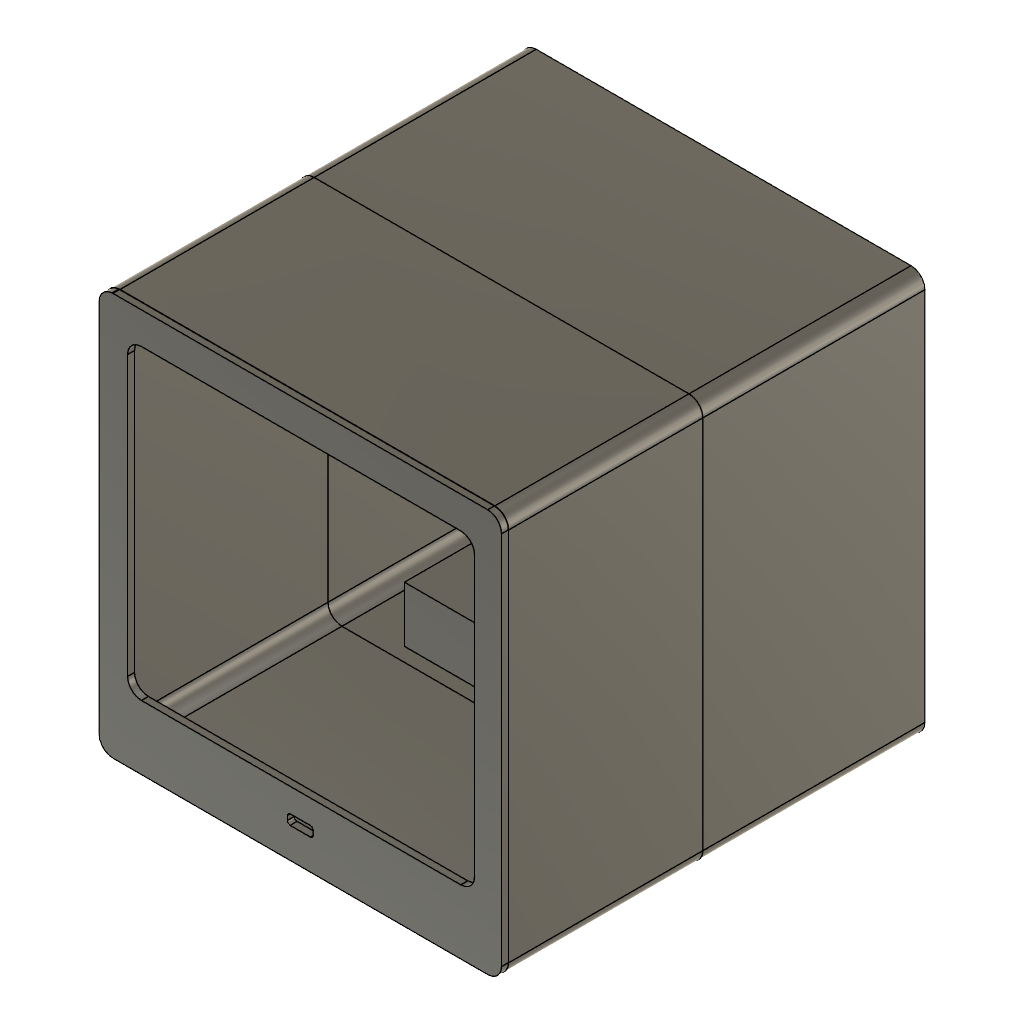
Fume Absorber (Autodesk Fusion 360 design; units mm, degrees)
part number: 2026-09-16-20-58-32-187
Autodesk Fusion 360 part; units mm, degrees
note: some values were not read from the file. Set by a fixed rule: which sketch regions a step uses.
(part 1 of 2)
sketch "Sketch2" plane through (0, 0, 0) normal (0, 1, 0) x (1, 0, 0)
  line L0 (-57.9957, -145.0372) -> (77.0043, -145.0372)
  line L1 (82.0043, -140.0372) -> (82.0043, -5.0372)
  line L2 (77.0043, -0.0372) -> (-57.9957, -0.0372)
  line L3 (-62.9957, -5.0372) -> (-62.9957, -140.0372)
  arc A0 (-62.9957, -140.0372) -> (-57.9957, -145.0372) centre (-57.9957, -140.0372) ccw
  arc A1 (77.0043, -145.0372) -> (82.0043, -140.0372) centre (77.0043, -140.0372) ccw
  arc A2 (82.0043, -5.0372) -> (77.0043, -0.0372) centre (77.0043, -5.0372) ccw
  arc A3 (-57.9957, -0.0372) -> (-62.9957, -5.0372) centre (-57.9957, -5.0372) ccw
  line L4 (-47.9957, -135.0372) -> (67.0043, -135.0372)
  line L5 (72.0043, -130.0372) -> (72.0043, -15.0372)
  line L6 (67.0043, -10.0372) -> (-47.9957, -10.0372)
  line L7 (-52.9957, -15.0372) -> (-52.9957, -130.0372)
  arc A4 (-52.9957, -130.0372) -> (-47.9957, -135.0372) centre (-47.9957, -130.0372) ccw
  arc A5 (67.0043, -135.0372) -> (72.0043, -130.0372) centre (67.0043, -130.0372) ccw
  arc A6 (72.0043, -15.0372) -> (67.0043, -10.0372) centre (67.0043, -15.0372) ccw
  arc A7 (-47.9957, -10.0372) -> (-52.9957, -15.0372) centre (-47.9957, -15.0372) ccw
  circle A8 centre (3.6938, -81.3062) radius 2.5
  circle A9 centre (10.5725, -75.1918) radius 2.5
  circle A10 centre (-66.3062, -141.3062) radius 2.5
  circle A11 centre (-59.4275, -135.1918) radius 2.5
  circle A12 centre (-59.3062, -141.3062) radius 2.5
  circle A13 centre (-52.4275, -135.1918) radius 2.5
  circle A14 centre (-52.3062, -141.3062) radius 2.5
  circle A15 centre (-45.4275, -135.1918) radius 2.5
  circle A16 centre (-45.3062, -141.3062) radius 2.5
  circle A17 centre (-38.4275, -135.1918) radius 2.5
  circle A18 centre (-38.3062, -141.3062) radius 2.5
  circle A19 centre (-31.4275, -135.1918) radius 2.5
  circle A20 centre (-31.3062, -141.3062) radius 2.5
  circle A21 centre (-24.4275, -135.1918) radius 2.5
  circle A22 centre (-24.3062, -141.3062) radius 2.5
  circle A23 centre (-17.4275, -135.1918) radius 2.5
  circle A24 centre (-17.3062, -141.3062) radius 2.5
  circle A25 centre (-10.4275, -135.1918) radius 2.5
  circle A26 centre (-10.3062, -141.3062) radius 2.5
  circle A27 centre (-3.4275, -135.1918) radius 2.5
  circle A28 centre (-3.3062, -141.3062) radius 2.5
  circle A29 centre (3.5725, -135.1918) radius 2.5
  circle A30 centre (3.6938, -141.3062) radius 2.5
  circle A31 centre (10.5725, -135.1918) radius 2.5
  circle A32 centre (10.6938, -141.3062) radius 2.5
  circle A33 centre (17.5725, -135.1918) radius 2.5
  circle A34 centre (17.6938, -141.3062) radius 2.5
  circle A35 centre (24.5725, -135.1918) radius 2.5
  circle A36 centre (24.6938, -141.3062) radius 2.5
  circle A37 centre (31.5725, -135.1918) radius 2.5
  circle A38 centre (31.6938, -141.3062) radius 2.5
  circle A39 centre (38.5725, -135.1918) radius 2.5
  circle A40 centre (38.6938, -141.3062) radius 2.5
  circle A41 centre (45.5725, -135.1918) radius 2.5
  circle A42 centre (45.6938, -141.3062) radius 2.5
  circle A43 centre (52.5725, -135.1918) radius 2.5
  circle A44 centre (52.6938, -141.3062) radius 2.5
  circle A45 centre (59.5725, -135.1918) radius 2.5
  circle A46 centre (59.6938, -141.3062) radius 2.5
  circle A47 centre (66.5725, -135.1918) radius 2.5
  circle A48 centre (66.6938, -141.3062) radius 2.5
  circle A49 centre (73.5725, -135.1918) radius 2.5
  circle A50 centre (73.6938, -141.3062) radius 2.5
  circle A51 centre (80.5725, -135.1918) radius 2.5
  circle A52 centre (-66.3062, -135.3062) radius 2.5
  circle A53 centre (-59.4275, -129.1918) radius 2.5
  circle A54 centre (-59.3062, -135.3062) radius 2.5
  circle A55 centre (-52.4275, -129.1918) radius 2.5
  circle A56 centre (-52.3062, -135.3062) radius 2.5
  circle A57 centre (-45.4275, -129.1918) radius 2.5
  circle A58 centre (-45.3062, -135.3062) radius 2.5
  circle A59 centre (-38.4275, -129.1918) radius 2.5
  circle A60 centre (-38.3062, -135.3062) radius 2.5
  circle A61 centre (-31.4275, -129.1918) radius 2.5
  circle A62 centre (-31.3062, -135.3062) radius 2.5
  circle A63 centre (-24.4275, -129.1918) radius 2.5
  circle A64 centre (-24.3062, -135.3062) radius 2.5
  circle A65 centre (-17.4275, -129.1918) radius 2.5
  circle A66 centre (-17.3062, -135.3062) radius 2.5
  circle A67 centre (-10.4275, -129.1918) radius 2.5
  circle A68 centre (-10.3062, -135.3062) radius 2.5
  circle A69 centre (-3.4275, -129.1918) radius 2.5
  circle A70 centre (-3.3062, -135.3062) radius 2.5
  circle A71 centre (3.5725, -129.1918) radius 2.5
  circle A72 centre (3.6938, -135.3062) radius 2.5
  circle A73 centre (10.5725, -129.1918) radius 2.5
  circle A74 centre (10.6938, -135.3062) radius 2.5
  circle A75 centre (17.5725, -129.1918) radius 2.5
  circle A76 centre (17.6938, -135.3062) radius 2.5
  circle A77 centre (24.5725, -129.1918) radius 2.5
  circle A78 centre (24.6938, -135.3062) radius 2.5
  circle A79 centre (31.5725, -129.1918) radius 2.5
  circle A80 centre (31.6938, -135.3062) radius 2.5
  circle A81 centre (38.5725, -129.1918) radius 2.5
  circle A82 centre (38.6938, -135.3062) radius 2.5
  circle A83 centre (45.5725, -129.1918) radius 2.5
  circle A84 centre (45.6938, -135.3062) radius 2.5
  circle A85 centre (52.5725, -129.1918) radius 2.5
  circle A86 centre (52.6938, -135.3062) radius 2.5
  circle A87 centre (59.5725, -129.1918) radius 2.5
  circle A88 centre (59.6938, -135.3062) radius 2.5
  circle A89 centre (66.5725, -129.1918) radius 2.5
  circle A90 centre (66.6938, -135.3062) radius 2.5
  circle A91 centre (73.5725, -129.1918) radius 2.5
  circle A92 centre (73.6938, -135.3062) radius 2.5
  circle A93 centre (80.5725, -129.1918) radius 2.5
  circle A94 centre (-66.3062, -129.3062) radius 2.5
  circle A95 centre (-59.4275, -123.1918) radius 2.5
  circle A96 centre (-59.3062, -129.3062) radius 2.5
  circle A97 centre (-52.4275, -123.1918) radius 2.5
  circle A98 centre (-52.3062, -129.3062) radius 2.5
  circle A99 centre (-45.4275, -123.1918) radius 2.5
  circle A100 centre (-45.3062, -129.3062) radius 2.5
  circle A101 centre (-38.4275, -123.1918) radius 2.5
  circle A102 centre (-38.3062, -129.3062) radius 2.5
  circle A103 centre (-31.4275, -123.1918) radius 2.5
  circle A104 centre (-31.3062, -129.3062) radius 2.5
  circle A105 centre (-24.4275, -123.1918) radius 2.5
  circle A106 centre (-24.3062, -129.3062) radius 2.5
  circle A107 centre (-17.4275, -123.1918) radius 2.5
  circle A108 centre (-17.3062, -129.3062) radius 2.5
  circle A109 centre (-10.4275, -123.1918) radius 2.5
  circle A110 centre (-10.3062, -129.3062) radius 2.5
  circle A111 centre (-3.4275, -123.1918) radius 2.5
  circle A112 centre (-3.3062, -129.3062) radius 2.5
  circle A113 centre (3.5725, -123.1918) radius 2.5
  circle A114 centre (3.6938, -129.3062) radius 2.5
  circle A115 centre (10.5725, -123.1918) radius 2.5
  circle A116 centre (10.6938, -129.3062) radius 2.5
  circle A117 centre (17.5725, -123.1918) radius 2.5
  circle A118 centre (17.6938, -129.3062) radius 2.5
  circle A119 centre (24.5725, -123.1918) radius 2.5
  circle A120 centre (24.6938, -129.3062) radius 2.5
  circle A121 centre (31.5725, -123.1918) radius 2.5
  circle A122 centre (31.6938, -129.3062) radius 2.5
  circle A123 centre (38.5725, -123.1918) radius 2.5
  circle A124 centre (38.6938, -129.3062) radius 2.5
  circle A125 centre (45.5725, -123.1918) radius 2.5
  circle A126 centre (45.6938, -129.3062) radius 2.5
  circle A127 centre (52.5725, -123.1918) radius 2.5
  circle A128 centre (52.6938, -129.3062) radius 2.5
  circle A129 centre (59.5725, -123.1918) radius 2.5
  circle A130 centre (59.6938, -129.3062) radius 2.5
  circle A131 centre (66.5725, -123.1918) radius 2.5
  circle A132 centre (66.6938, -129.3062) radius 2.5
  circle A133 centre (73.5725, -123.1918) radius 2.5
  circle A134 centre (73.6938, -129.3062) radius 2.5
  circle A135 centre (80.5725, -123.1918) radius 2.5
  circle A136 centre (-66.3062, -123.3062) radius 2.5
  circle A137 centre (-59.4275, -117.1918) radius 2.5
  circle A138 centre (-59.3062, -123.3062) radius 2.5
  circle A139 centre (-52.4275, -117.1918) radius 2.5
  circle A140 centre (-52.3062, -123.3062) radius 2.5
  circle A141 centre (-45.4275, -117.1918) radius 2.5
  circle A142 centre (-45.3062, -123.3062) radius 2.5
  circle A143 centre (-38.4275, -117.1918) radius 2.5
  circle A144 centre (-38.3062, -123.3062) radius 2.5
  circle A145 centre (-31.4275, -117.1918) radius 2.5
  circle A146 centre (-31.3062, -123.3062) radius 2.5
  circle A147 centre (-24.4275, -117.1918) radius 2.5
  circle A148 centre (-24.3062, -123.3062) radius 2.5
  circle A149 centre (-17.4275, -117.1918) radius 2.5
  circle A150 centre (-17.3062, -123.3062) radius 2.5
  circle A151 centre (-10.4275, -117.1918) radius 2.5
  circle A152 centre (-10.3062, -123.3062) radius 2.5
  circle A153 centre (-3.4275, -117.1918) radius 2.5
  circle A154 centre (-3.3062, -123.3062) radius 2.5
  circle A155 centre (3.5725, -117.1918) radius 2.5
  circle A156 centre (3.6938, -123.3062) radius 2.5
  circle A157 centre (10.5725, -117.1918) radius 2.5
  circle A158 centre (10.6938, -123.3062) radius 2.5
  circle A159 centre (17.5725, -117.1918) radius 2.5
  circle A160 centre (17.6938, -123.3062) radius 2.5
  circle A161 centre (24.5725, -117.1918) radius 2.5
  circle A162 centre (24.6938, -123.3062) radius 2.5
  circle A163 centre (31.5725, -117.1918) radius 2.5
  circle A164 centre (31.6938, -123.3062) radius 2.5
  circle A165 centre (38.5725, -117.1918) radius 2.5
  circle A166 centre (38.6938, -123.3062) radius 2.5
  circle A167 centre (45.5725, -117.1918) radius 2.5
  circle A168 centre (45.6938, -123.3062) radius 2.5
  circle A169 centre (52.5725, -117.1918) radius 2.5
  circle A170 centre (52.6938, -123.3062) radius 2.5
  circle A171 centre (59.5725, -117.1918) radius 2.5
  circle A172 centre (59.6938, -123.3062) radius 2.5
  circle A173 centre (66.5725, -117.1918) radius 2.5
  circle A174 centre (66.6938, -123.3062) radius 2.5
  circle A175 centre (73.5725, -117.1918) radius 2.5
  circle A176 centre (73.6938, -123.3062) radius 2.5
  circle A177 centre (80.5725, -117.1918) radius 2.5
  circle A178 centre (-66.3062, -117.3062) radius 2.5
  circle A179 centre (-59.4275, -111.1918) radius 2.5
  circle A180 centre (-59.3062, -117.3062) radius 2.5
  circle A181 centre (-52.4275, -111.1918) radius 2.5
  circle A182 centre (-52.3062, -117.3062) radius 2.5
  circle A183 centre (-45.4275, -111.1918) radius 2.5
  circle A184 centre (-45.3062, -117.3062) radius 2.5
  circle A185 centre (-38.4275, -111.1918) radius 2.5
  circle A186 centre (-38.3062, -117.3062) radius 2.5
  circle A187 centre (-31.4275, -111.1918) radius 2.5
  circle A188 centre (-31.3062, -117.3062) radius 2.5
  circle A189 centre (-24.4275, -111.1918) radius 2.5
  circle A190 centre (-24.3062, -117.3062) radius 2.5
  circle A191 centre (-17.4275, -111.1918) radius 2.5
  circle A192 centre (-17.3062, -117.3062) radius 2.5
  circle A193 centre (-10.4275, -111.1918) radius 2.5
  circle A194 centre (-10.3062, -117.3062) radius 2.5
  circle A195 centre (-3.4275, -111.1918) radius 2.5
  circle A196 centre (-3.3062, -117.3062) radius 2.5
  circle A197 centre (3.5725, -111.1918) radius 2.5
  circle A198 centre (3.6938, -117.3062) radius 2.5
  circle A199 centre (10.5725, -111.1918) radius 2.5
  circle A200 centre (10.6938, -117.3062) radius 2.5
  circle A201 centre (17.5725, -111.1918) radius 2.5
  circle A202 centre (17.6938, -117.3062) radius 2.5
  circle A203 centre (24.5725, -111.1918) radius 2.5
  circle A204 centre (24.6938, -117.3062) radius 2.5
  circle A205 centre (31.5725, -111.1918) radius 2.5
  circle A206 centre (31.6938, -117.3062) radius 2.5
  circle A207 centre (38.5725, -111.1918) radius 2.5
  circle A208 centre (38.6938, -117.3062) radius 2.5
  circle A209 centre (45.5725, -111.1918) radius 2.5
  circle A210 centre (45.6938, -117.3062) radius 2.5
  circle A211 centre (52.5725, -111.1918) radius 2.5
  circle A212 centre (52.6938, -117.3062) radius 2.5
  circle A213 centre (59.5725, -111.1918) radius 2.5
  circle A214 centre (59.6938, -117.3062) radius 2.5
  circle A215 centre (66.5725, -111.1918) radius 2.5
  circle A216 centre (66.6938, -117.3062) radius 2.5
  circle A217 centre (73.5725, -111.1918) radius 2.5
  circle A218 centre (73.6938, -117.3062) radius 2.5
  circle A219 centre (80.5725, -111.1918) radius 2.5
  circle A220 centre (-66.3062, -111.3062) radius 2.5
  circle A221 centre (-59.4275, -105.1918) radius 2.5
  circle A222 centre (-59.3062, -111.3062) radius 2.5
  circle A223 centre (-52.4275, -105.1918) radius 2.5
  circle A224 centre (-52.3062, -111.3062) radius 2.5
  circle A225 centre (-45.4275, -105.1918) radius 2.5
  circle A226 centre (-45.3062, -111.3062) radius 2.5
  circle A227 centre (-38.4275, -105.1918) radius 2.5
  circle A228 centre (-38.3062, -111.3062) radius 2.5
  circle A229 centre (-31.4275, -105.1918) radius 2.5
  circle A230 centre (-31.3062, -111.3062) radius 2.5
  circle A231 centre (-24.4275, -105.1918) radius 2.5
  circle A232 centre (-24.3062, -111.3062) radius 2.5
  circle A233 centre (-17.4275, -105.1918) radius 2.5
  circle A234 centre (-17.3062, -111.3062) radius 2.5
  circle A235 centre (-10.4275, -105.1918) radius 2.5
  circle A236 centre (-10.3062, -111.3062) radius 2.5
  circle A237 centre (-3.4275, -105.1918) radius 2.5
  circle A238 centre (-3.3062, -111.3062) radius 2.5
  circle A239 centre (3.5725, -105.1918) radius 2.5
  circle A240 centre (3.6938, -111.3062) radius 2.5
  circle A241 centre (10.5725, -105.1918) radius 2.5
  circle A242 centre (10.6938, -111.3062) radius 2.5
  circle A243 centre (17.5725, -105.1918) radius 2.5
  circle A244 centre (17.6938, -111.3062) radius 2.5
  circle A245 centre (24.5725, -105.1918) radius 2.5
  circle A246 centre (24.6938, -111.3062) radius 2.5
  circle A247 centre (31.5725, -105.1918) radius 2.5
  circle A248 centre (31.6938, -111.3062) radius 2.5
  circle A249 centre (38.5725, -105.1918) radius 2.5
  circle A250 centre (38.6938, -111.3062) radius 2.5
  circle A251 centre (45.5725, -105.1918) radius 2.5
  circle A252 centre (45.6938, -111.3062) radius 2.5
  circle A253 centre (52.5725, -105.1918) radius 2.5
  circle A254 centre (52.6938, -111.3062) radius 2.5
  circle A255 centre (59.5725, -105.1918) radius 2.5
  circle A256 centre (59.6938, -111.3062) radius 2.5
  circle A257 centre (66.5725, -105.1918) radius 2.5
  circle A258 centre (66.6938, -111.3062) radius 2.5
  circle A259 centre (73.5725, -105.1918) radius 2.5
  circle A260 centre (73.6938, -111.3062) radius 2.5
  circle A261 centre (80.5725, -105.1918) radius 2.5
  circle A262 centre (-66.3062, -105.3062) radius 2.5
  circle A263 centre (-59.4275, -99.1918) radius 2.5
  circle A264 centre (-59.3062, -105.3062) radius 2.5
  circle A265 centre (-52.4275, -99.1918) radius 2.5
  circle A266 centre (-52.3062, -105.3062) radius 2.5
  circle A267 centre (-45.4275, -99.1918) radius 2.5
  circle A268 centre (-45.3062, -105.3062) radius 2.5
  circle A269 centre (-38.4275, -99.1918) radius 2.5
  circle A270 centre (-38.3062, -105.3062) radius 2.5
  circle A271 centre (-31.4275, -99.1918) radius 2.5
  circle A272 centre (-31.3062, -105.3062) radius 2.5
  circle A273 centre (-24.4275, -99.1918) radius 2.5
  circle A274 centre (-24.3062, -105.3062) radius 2.5
  circle A275 centre (-17.4275, -99.1918) radius 2.5
  circle A276 centre (-17.3062, -105.3062) radius 2.5
  circle A277 centre (-10.4275, -99.1918) radius 2.5
  circle A278 centre (-10.3062, -105.3062) radius 2.5
  circle A279 centre (-3.4275, -99.1918) radius 2.5
  circle A280 centre (-3.3062, -105.3062) radius 2.5
  circle A281 centre (3.5725, -99.1918) radius 2.5
  circle A282 centre (3.6938, -105.3062) radius 2.5
  circle A283 centre (10.5725, -99.1918) radius 2.5
  circle A284 centre (10.6938, -105.3062) radius 2.5
  circle A285 centre (17.5725, -99.1918) radius 2.5
  circle A286 centre (17.6938, -105.3062) radius 2.5
  circle A287 centre (24.5725, -99.1918) radius 2.5
  circle A288 centre (24.6938, -105.3062) radius 2.5
  circle A289 centre (31.5725, -99.1918) radius 2.5
  circle A290 centre (31.6938, -105.3062) radius 2.5
  circle A291 centre (38.5725, -99.1918) radius 2.5
  circle A292 centre (38.6938, -105.3062) radius 2.5
  circle A293 centre (45.5725, -99.1918) radius 2.5
  circle A294 centre (45.6938, -105.3062) radius 2.5
  circle A295 centre (52.5725, -99.1918) radius 2.5
  circle A296 centre (52.6938, -105.3062) radius 2.5
  circle A297 centre (59.5725, -99.1918) radius 2.5
  circle A298 centre (59.6938, -105.3062) radius 2.5
  circle A299 centre (66.5725, -99.1918) radius 2.5
  circle A300 centre (66.6938, -105.3062) radius 2.5
  circle A301 centre (73.5725, -99.1918) radius 2.5
  circle A302 centre (73.6938, -105.3062) radius 2.5
  circle A303 centre (80.5725, -99.1918) radius 2.5
  circle A304 centre (-66.3062, -99.3062) radius 2.5
  circle A305 centre (-59.4275, -93.1918) radius 2.5
  circle A306 centre (-59.3062, -99.3062) radius 2.5
  circle A307 centre (-52.4275, -93.1918) radius 2.5
  circle A308 centre (-52.3062, -99.3062) radius 2.5
  circle A309 centre (-45.4275, -93.1918) radius 2.5
  circle A310 centre (-45.3062, -99.3062) radius 2.5
  circle A311 centre (-38.4275, -93.1918) radius 2.5
  circle A312 centre (-38.3062, -99.3062) radius 2.5
  circle A313 centre (-31.4275, -93.1918) radius 2.5
  circle A314 centre (-31.3062, -99.3062) radius 2.5
  circle A315 centre (-24.4275, -93.1918) radius 2.5
  circle A316 centre (-24.3062, -99.3062) radius 2.5
  circle A317 centre (-17.4275, -93.1918) radius 2.5
  circle A318 centre (-17.3062, -99.3062) radius 2.5
  circle A319 centre (-10.4275, -93.1918) radius 2.5
  circle A320 centre (-10.3062, -99.3062) radius 2.5
  circle A321 centre (-3.4275, -93.1918) radius 2.5
  circle A322 centre (-3.3062, -99.3062) radius 2.5
  circle A323 centre (3.5725, -93.1918) radius 2.5
  circle A324 centre (3.6938, -99.3062) radius 2.5
  circle A325 centre (10.5725, -93.1918) radius 2.5
  circle A326 centre (10.6938, -99.3062) radius 2.5
  circle A327 centre (17.5725, -93.1918) radius 2.5
  circle A328 centre (17.6938, -99.3062) radius 2.5
  circle A329 centre (24.5725, -93.1918) radius 2.5
  circle A330 centre (24.6938, -99.3062) radius 2.5
  circle A331 centre (31.5725, -93.1918) radius 2.5
  circle A332 centre (31.6938, -99.3062) radius 2.5
  circle A333 centre (38.5725, -93.1918) radius 2.5
  circle A334 centre (38.6938, -99.3062) radius 2.5
  circle A335 centre (45.5725, -93.1918) radius 2.5
  circle A336 centre (45.6938, -99.3062) radius 2.5
  circle A337 centre (52.5725, -93.1918) radius 2.5
  circle A338 centre (52.6938, -99.3062) radius 2.5
  circle A339 centre (59.5725, -93.1918) radius 2.5
  circle A340 centre (59.6938, -99.3062) radius 2.5
  circle A341 centre (66.5725, -93.1918) radius 2.5
  circle A342 centre (66.6938, -99.3062) radius 2.5
  circle A343 centre (73.5725, -93.1918) radius 2.5
  circle A344 centre (73.6938, -99.3062) radius 2.5
  circle A345 centre (80.5725, -93.1918) radius 2.5
  circle A346 centre (-66.3062, -93.3062) radius 2.5
  circle A347 centre (-59.4275, -87.1918) radius 2.5
  circle A348 centre (-59.3062, -93.3062) radius 2.5
  circle A349 centre (-52.4275, -87.1918) radius 2.5
  circle A350 centre (-52.3062, -93.3062) radius 2.5
  circle A351 centre (-45.4275, -87.1918) radius 2.5
  circle A352 centre (-45.3062, -93.3062) radius 2.5
  circle A353 centre (-38.4275, -87.1918) radius 2.5
  circle A354 centre (-38.3062, -93.3062) radius 2.5
  circle A355 centre (-31.4275, -87.1918) radius 2.5
  circle A356 centre (-31.3062, -93.3062) radius 2.5
  circle A357 centre (-24.4275, -87.1918) radius 2.5
  circle A358 centre (-24.3062, -93.3062) radius 2.5
  circle A359 centre (-17.4275, -87.1918) radius 2.5
  circle A360 centre (-17.3062, -93.3062) radius 2.5
  circle A361 centre (-10.4275, -87.1918) radius 2.5
  circle A362 centre (-10.3062, -93.3062) radius 2.5
  circle A363 centre (-3.4275, -87.1918) radius 2.5
  circle A364 centre (-3.3062, -93.3062) radius 2.5
  circle A365 centre (3.5725, -87.1918) radius 2.5
  circle A366 centre (3.6938, -93.3062) radius 2.5
  circle A367 centre (10.5725, -87.1918) radius 2.5
  circle A368 centre (10.6938, -93.3062) radius 2.5
  circle A369 centre (17.5725, -87.1918) radius 2.5
  circle A370 centre (17.6938, -93.3062) radius 2.5
  circle A371 centre (24.5725, -87.1918) radius 2.5
  circle A372 centre (24.6938, -93.3062) radius 2.5
  circle A373 centre (31.5725, -87.1918) radius 2.5
  circle A374 centre (31.6938, -93.3062) radius 2.5
  circle A375 centre (38.5725, -87.1918) radius 2.5
  circle A376 centre (38.6938, -93.3062) radius 2.5
  circle A377 centre (45.5725, -87.1918) radius 2.5
  circle A378 centre (45.6938, -93.3062) radius 2.5
  circle A379 centre (52.5725, -87.1918) radius 2.5
  circle A380 centre (52.6938, -93.3062) radius 2.5
  circle A381 centre (59.5725, -87.1918) radius 2.5
  circle A382 centre (59.6938, -93.3062) radius 2.5
  circle A383 centre (66.5725, -87.1918) radius 2.5
  circle A384 centre (66.6938, -93.3062) radius 2.5
  circle A385 centre (73.5725, -87.1918) radius 2.5
  circle A386 centre (73.6938, -93.3062) radius 2.5
  circle A387 centre (80.5725, -87.1918) radius 2.5
  circle A388 centre (-66.3062, -87.3062) radius 2.5
  circle A389 centre (-59.4275, -81.1918) radius 2.5
  circle A390 centre (-59.3062, -87.3062) radius 2.5
  circle A391 centre (-52.4275, -81.1918) radius 2.5
  circle A392 centre (-52.3062, -87.3062) radius 2.5
  circle A393 centre (-45.4275, -81.1918) radius 2.5
  circle A394 centre (-45.3062, -87.3062) radius 2.5
  circle A395 centre (-38.4275, -81.1918) radius 2.5
  circle A396 centre (-38.3062, -87.3062) radius 2.5
  circle A397 centre (-31.4275, -81.1918) radius 2.5
  circle A398 centre (-31.3062, -87.3062) radius 2.5
  circle A399 centre (-24.4275, -81.1918) radius 2.5
  circle A400 centre (-24.3062, -87.3062) radius 2.5
  circle A401 centre (-17.4275, -81.1918) radius 2.5
  circle A402 centre (-17.3062, -87.3062) radius 2.5
  circle A403 centre (-10.4275, -81.1918) radius 2.5
  circle A404 centre (-10.3062, -87.3062) radius 2.5
  circle A405 centre (-3.4275, -81.1918) radius 2.5
  circle A406 centre (-3.3062, -87.3062) radius 2.5
  circle A407 centre (3.5725, -81.1918) radius 2.5
  circle A408 centre (3.6938, -87.3062) radius 2.5
  circle A409 centre (10.5725, -81.1918) radius 2.5
  circle A410 centre (10.6938, -87.3062) radius 2.5
  circle A411 centre (17.5725, -81.1918) radius 2.5
  circle A412 centre (17.6938, -87.3062) radius 2.5
  circle A413 centre (24.5725, -81.1918) radius 2.5
  circle A414 centre (24.6938, -87.3062) radius 2.5
  circle A415 centre (31.5725, -81.1918) radius 2.5
  circle A416 centre (31.6938, -87.3062) radius 2.5
  circle A417 centre (38.5725, -81.1918) radius 2.5
  circle A418 centre (38.6938, -87.3062) radius 2.5
  circle A419 centre (45.5725, -81.1918) radius 2.5
  circle A420 centre (45.6938, -87.3062) radius 2.5
  circle A421 centre (52.5725, -81.1918) radius 2.5
  circle A422 centre (52.6938, -87.3062) radius 2.5
  circle A423 centre (59.5725, -81.1918) radius 2.5
  circle A424 centre (59.6938, -87.3062) radius 2.5
  circle A425 centre (66.5725, -81.1918) radius 2.5
  circle A426 centre (66.6938, -87.3062) radius 2.5
  circle A427 centre (73.5725, -81.1918) radius 2.5
  circle A428 centre (73.6938, -87.3062) radius 2.5
  circle A429 centre (80.5725, -81.1918) radius 2.5
  circle A430 centre (-66.3062, -81.3062) radius 2.5
  circle A431 centre (-59.4275, -75.1918) radius 2.5
  circle A432 centre (-59.3062, -81.3062) radius 2.5
  circle A433 centre (-52.4275, -75.1918) radius 2.5
  circle A434 centre (-52.3062, -81.3062) radius 2.5
  circle A435 centre (-45.4275, -75.1918) radius 2.5
  circle A436 centre (-45.3062, -81.3062) radius 2.5
  circle A437 centre (-38.4275, -75.1918) radius 2.5
  circle A438 centre (-38.3062, -81.3062) radius 2.5
  circle A439 centre (-31.4275, -75.1918) radius 2.5
  circle A440 centre (-31.3062, -81.3062) radius 2.5
  circle A441 centre (-24.4275, -75.1918) radius 2.5
  circle A442 centre (-24.3062, -81.3062) radius 2.5
  circle A443 centre (-17.4275, -75.1918) radius 2.5
  circle A444 centre (-17.3062, -81.3062) radius 2.5
  circle A445 centre (-10.4275, -75.1918) radius 2.5
  circle A446 centre (-10.3062, -81.3062) radius 2.5
  circle A447 centre (-3.4275, -75.1918) radius 2.5
  circle A448 centre (-3.3062, -81.3062) radius 2.5
  circle A449 centre (3.5725, -75.1918) radius 2.5
  circle A450 centre (10.6938, -81.3062) radius 2.5
  circle A451 centre (17.5725, -75.1918) radius 2.5
  circle A452 centre (17.6938, -81.3062) radius 2.5
  circle A453 centre (24.5725, -75.1918) radius 2.5
  circle A454 centre (24.6938, -81.3062) radius 2.5
  circle A455 centre (31.5725, -75.1918) radius 2.5
  circle A456 centre (31.6938, -81.3062) radius 2.5
  circle A457 centre (38.5725, -75.1918) radius 2.5
  circle A458 centre (38.6938, -81.3062) radius 2.5
  circle A459 centre (45.5725, -75.1918) radius 2.5
  circle A460 centre (45.6938, -81.3062) radius 2.5
  circle A461 centre (52.5725, -75.1918) radius 2.5
  circle A462 centre (52.6938, -81.3062) radius 2.5
  circle A463 centre (59.5725, -75.1918) radius 2.5
  circle A464 centre (59.6938, -81.3062) radius 2.5
  circle A465 centre (66.5725, -75.1918) radius 2.5
  circle A466 centre (66.6938, -81.3062) radius 2.5
  circle A467 centre (73.5725, -75.1918) radius 2.5
  circle A468 centre (73.6938, -81.3062) radius 2.5
  circle A469 centre (80.5725, -75.1918) radius 2.5
  circle A470 centre (-66.3062, -75.3062) radius 2.5
  circle A471 centre (-59.4275, -69.1918) radius 2.5
  circle A472 centre (-59.3062, -75.3062) radius 2.5
  circle A473 centre (-52.4275, -69.1918) radius 2.5
  circle A474 centre (-52.3062, -75.3062) radius 2.5
  circle A475 centre (-45.4275, -69.1918) radius 2.5
  circle A476 centre (-45.3062, -75.3062) radius 2.5
  circle A477 centre (-38.4275, -69.1918) radius 2.5
  circle A478 centre (-38.3062, -75.3062) radius 2.5
  circle A479 centre (-31.4275, -69.1918) radius 2.5
  circle A480 centre (-31.3062, -75.3062) radius 2.5
  circle A481 centre (-24.4275, -69.1918) radius 2.5
  circle A482 centre (-24.3062, -75.3062) radius 2.5
  circle A483 centre (-17.4275, -69.1918) radius 2.5
  circle A484 centre (-17.3062, -75.3062) radius 2.5
  circle A485 centre (-10.4275, -69.1918) radius 2.5
  circle A486 centre (-10.3062, -75.3062) radius 2.5
  circle A487 centre (-3.4275, -69.1918) radius 2.5
  circle A488 centre (-3.3062, -75.3062) radius 2.5
  circle A489 centre (3.5725, -69.1918) radius 2.5
  circle A490 centre (3.6938, -75.3062) radius 2.5
  circle A491 centre (10.5725, -69.1918) radius 2.5
  circle A492 centre (10.6938, -75.3062) radius 2.5
  circle A493 centre (17.5725, -69.1918) radius 2.5
  circle A494 centre (17.6938, -75.3062) radius 2.5
  circle A495 centre (24.5725, -69.1918) radius 2.5
  circle A496 centre (24.6938, -75.3062) radius 2.5
  circle A497 centre (31.5725, -69.1918) radius 2.5
  circle A498 centre (31.6938, -75.3062) radius 2.5
  circle A499 centre (38.5725, -69.1918) radius 2.5
  circle A500 centre (38.6938, -75.3062) radius 2.5
  circle A501 centre (45.5725, -69.1918) radius 2.5
  circle A502 centre (45.6938, -75.3062) radius 2.5
  circle A503 centre (52.5725, -69.1918) radius 2.5
  circle A504 centre (52.6938, -75.3062) radius 2.5
  circle A505 centre (59.5725, -69.1918) radius 2.5
  circle A506 centre (59.6938, -75.3062) radius 2.5
  circle A507 centre (66.5725, -69.1918) radius 2.5
  circle A508 centre (66.6938, -75.3062) radius 2.5
  circle A509 centre (73.5725, -69.1918) radius 2.5
  circle A510 centre (73.6938, -75.3062) radius 2.5
  circle A511 centre (80.5725, -69.1918) radius 2.5
  circle A512 centre (-66.3062, -69.3062) radius 2.5
  circle A513 centre (-59.4275, -63.1918) radius 2.5
  circle A514 centre (-59.3062, -69.3062) radius 2.5
  circle A515 centre (-52.4275, -63.1918) radius 2.5
  circle A516 centre (-52.3062, -69.3062) radius 2.5
  circle A517 centre (-45.4275, -63.1918) radius 2.5
  circle A518 centre (-45.3062, -69.3062) radius 2.5
  circle A519 centre (-38.4275, -63.1918) radius 2.5
  circle A520 centre (-38.3062, -69.3062) radius 2.5
  circle A521 centre (-31.4275, -63.1918) radius 2.5
  circle A522 centre (-31.3062, -69.3062) radius 2.5
  circle A523 centre (-24.4275, -63.1918) radius 2.5
  circle A524 centre (-24.3062, -69.3062) radius 2.5
  circle A525 centre (-17.4275, -63.1918) radius 2.5
  circle A526 centre (-17.3062, -69.3062) radius 2.5
  circle A527 centre (-10.4275, -63.1918) radius 2.5
  circle A528 centre (-10.3062, -69.3062) radius 2.5
  circle A529 centre (-3.4275, -63.1918) radius 2.5
  circle A530 centre (-3.3062, -69.3062) radius 2.5
  circle A531 centre (3.5725, -63.1918) radius 2.5
  circle A532 centre (3.6938, -69.3062) radius 2.5
  circle A533 centre (10.5725, -63.1918) radius 2.5
  circle A534 centre (10.6938, -69.3062) radius 2.5
  circle A535 centre (17.5725, -63.1918) radius 2.5
  circle A536 centre (17.6938, -69.3062) radius 2.5
  circle A537 centre (24.5725, -63.1918) radius 2.5
  circle A538 centre (24.6938, -69.3062) radius 2.5
  circle A539 centre (31.5725, -63.1918) radius 2.5
  circle A540 centre (31.6938, -69.3062) radius 2.5
  circle A541 centre (38.5725, -63.1918) radius 2.5
  circle A542 centre (38.6938, -69.3062) radius 2.5
  circle A543 centre (45.5725, -63.1918) radius 2.5
  circle A544 centre (45.6938, -69.3062) radius 2.5
  circle A545 centre (52.5725, -63.1918) radius 2.5
  circle A546 centre (52.6938, -69.3062) radius 2.5
  circle A547 centre (59.5725, -63.1918) radius 2.5
  circle A548 centre (59.6938, -69.3062) radius 2.5
  circle A549 centre (66.5725, -63.1918) radius 2.5
  circle A550 centre (66.6938, -69.3062) radius 2.5
  circle A551 centre (73.5725, -63.1918) radius 2.5
  circle A552 centre (73.6938, -69.3062) radius 2.5
  circle A553 centre (80.5725, -63.1918) radius 2.5
  circle A554 centre (-66.3062, -63.3062) radius 2.5
  circle A555 centre (-59.4275, -57.1918) radius 2.5
  circle A556 centre (-59.3062, -63.3062) radius 2.5
  circle A557 centre (-52.4275, -57.1918) radius 2.5
  circle A558 centre (-52.3062, -63.3062) radius 2.5
  circle A559 centre (-45.4275, -57.1918) radius 2.5
  circle A560 centre (-45.3062, -63.3062) radius 2.5
  circle A561 centre (-38.4275, -57.1918) radius 2.5
  circle A562 centre (-38.3062, -63.3062) radius 2.5
  circle A563 centre (-31.4275, -57.1918) radius 2.5
  circle A564 centre (-31.3062, -63.3062) radius 2.5
  circle A565 centre (-24.4275, -57.1918) radius 2.5
  circle A566 centre (-24.3062, -63.3062) radius 2.5
  circle A567 centre (-17.4275, -57.1918) radius 2.5
  circle A568 centre (-17.3062, -63.3062) radius 2.5
  circle A569 centre (-10.4275, -57.1918) radius 2.5
  circle A570 centre (-10.3062, -63.3062) radius 2.5
  circle A571 centre (-3.4275, -57.1918) radius 2.5
  circle A572 centre (-3.3062, -63.3062) radius 2.5
  circle A573 centre (3.5725, -57.1918) radius 2.5
  circle A574 centre (3.6938, -63.3062) radius 2.5
  circle A575 centre (10.5725, -57.1918) radius 2.5
  circle A576 centre (10.6938, -63.3062) radius 2.5
  circle A577 centre (17.5725, -57.1918) radius 2.5
  circle A578 centre (17.6938, -63.3062) radius 2.5
  circle A579 centre (24.5725, -57.1918) radius 2.5
  circle A580 centre (24.6938, -63.3062) radius 2.5
  circle A581 centre (31.5725, -57.1918) radius 2.5
  circle A582 centre (31.6938, -63.3062) radius 2.5
  circle A583 centre (38.5725, -57.1918) radius 2.5
  circle A584 centre (38.6938, -63.3062) radius 2.5
  circle A585 centre (45.5725, -57.1918) radius 2.5
  circle A586 centre (45.6938, -63.3062) radius 2.5
  circle A587 centre (52.5725, -57.1918) radius 2.5
  circle A588 centre (52.6938, -63.3062) radius 2.5
  circle A589 centre (59.5725, -57.1918) radius 2.5
  circle A590 centre (59.6938, -63.3062) radius 2.5
  circle A591 centre (66.5725, -57.1918) radius 2.5
  circle A592 centre (66.6938, -63.3062) radius 2.5
  circle A593 centre (73.5725, -57.1918) radius 2.5
  circle A594 centre (73.6938, -63.3062) radius 2.5
  circle A595 centre (80.5725, -57.1918) radius 2.5
  circle A596 centre (-66.3062, -57.3062) radius 2.5
  circle A597 centre (-59.4275, -51.1918) radius 2.5
  circle A598 centre (-59.3062, -57.3062) radius 2.5
  circle A599 centre (-52.4275, -51.1918) radius 2.5
  circle A600 centre (-52.3062, -57.3062) radius 2.5
  circle A601 centre (-45.4275, -51.1918) radius 2.5
  circle A602 centre (-45.3062, -57.3062) radius 2.5
  circle A603 centre (-38.4275, -51.1918) radius 2.5
  circle A604 centre (-38.3062, -57.3062) radius 2.5
  circle A605 centre (-31.4275, -51.1918) radius 2.5
  circle A606 centre (-31.3062, -57.3062) radius 2.5
  circle A607 centre (-24.4275, -51.1918) radius 2.5
  circle A608 centre (-24.3062, -57.3062) radius 2.5
  circle A609 centre (-17.4275, -51.1918) radius 2.5
  circle A610 centre (-17.3062, -57.3062) radius 2.5
  circle A611 centre (-10.4275, -51.1918) radius 2.5
  circle A612 centre (-10.3062, -57.3062) radius 2.5
  circle A613 centre (-3.4275, -51.1918) radius 2.5
  circle A614 centre (-3.3062, -57.3062) radius 2.5
  circle A615 centre (3.5725, -51.1918) radius 2.5
  circle A616 centre (3.6938, -57.3062) radius 2.5
  circle A617 centre (10.5725, -51.1918) radius 2.5
  circle A618 centre (10.6938, -57.3062) radius 2.5
  circle A619 centre (17.5725, -51.1918) radius 2.5
  circle A620 centre (17.6938, -57.3062) radius 2.5
  circle A621 centre (24.5725, -51.1918) radius 2.5
  circle A622 centre (24.6938, -57.3062) radius 2.5
  circle A623 centre (31.5725, -51.1918) radius 2.5
  circle A624 centre (31.6938, -57.3062) radius 2.5
  circle A625 centre (38.5725, -51.1918) radius 2.5
  circle A626 centre (38.6938, -57.3062) radius 2.5
  circle A627 centre (45.5725, -51.1918) radius 2.5
  circle A628 centre (45.6938, -57.3062) radius 2.5
  circle A629 centre (52.5725, -51.1918) radius 2.5
  circle A630 centre (52.6938, -57.3062) radius 2.5
  circle A631 centre (59.5725, -51.1918) radius 2.5
  circle A632 centre (59.6938, -57.3062) radius 2.5
  circle A633 centre (66.5725, -51.1918) radius 2.5
  circle A634 centre (66.6938, -57.3062) radius 2.5
  circle A635 centre (73.5725, -51.1918) radius 2.5
  circle A636 centre (73.6938, -57.3062) radius 2.5
  circle A637 centre (80.5725, -51.1918) radius 2.5
  circle A638 centre (-66.3062, -51.3062) radius 2.5
  circle A639 centre (-59.4275, -45.1918) radius 2.5
  circle A640 centre (-59.3062, -51.3062) radius 2.5
  circle A641 centre (-52.4275, -45.1918) radius 2.5
  circle A642 centre (-52.3062, -51.3062) radius 2.5
  circle A643 centre (-45.4275, -45.1918) radius 2.5
  circle A644 centre (-45.3062, -51.3062) radius 2.5
  circle A645 centre (-38.4275, -45.1918) radius 2.5
  circle A646 centre (-38.3062, -51.3062) radius 2.5
  circle A647 centre (-31.4275, -45.1918) radius 2.5
  circle A648 centre (-31.3062, -51.3062) radius 2.5
  circle A649 centre (-24.4275, -45.1918) radius 2.5
  circle A650 centre (-24.3062, -51.3062) radius 2.5
  circle A651 centre (-17.4275, -45.1918) radius 2.5
  circle A652 centre (-17.3062, -51.3062) radius 2.5
  circle A653 centre (-10.4275, -45.1918) radius 2.5
  circle A654 centre (-10.3062, -51.3062) radius 2.5
  circle A655 centre (-3.4275, -45.1918) radius 2.5
  circle A656 centre (-3.3062, -51.3062) radius 2.5
  circle A657 centre (3.5725, -45.1918) radius 2.5
  circle A658 centre (3.6938, -51.3062) radius 2.5
  circle A659 centre (10.5725, -45.1918) radius 2.5
  circle A660 centre (10.6938, -51.3062) radius 2.5
  circle A661 centre (17.5725, -45.1918) radius 2.5
  circle A662 centre (17.6938, -51.3062) radius 2.5
  circle A663 centre (24.5725, -45.1918) radius 2.5
  circle A664 centre (24.6938, -51.3062) radius 2.5
  circle A665 centre (31.5725, -45.1918) radius 2.5
  circle A666 centre (31.6938, -51.3062) radius 2.5
  circle A667 centre (38.5725, -45.1918) radius 2.5
  circle A668 centre (38.6938, -51.3062) radius 2.5
  circle A669 centre (45.5725, -45.1918) radius 2.5
  circle A670 centre (45.6938, -51.3062) radius 2.5
  circle A671 centre (52.5725, -45.1918) radius 2.5
  circle A672 centre (52.6938, -51.3062) radius 2.5
  circle A673 centre (59.5725, -45.1918) radius 2.5
  circle A674 centre (59.6938, -51.3062) radius 2.5
  circle A675 centre (66.5725, -45.1918) radius 2.5
  circle A676 centre (66.6938, -51.3062) radius 2.5
  circle A677 centre (73.5725, -45.1918) radius 2.5
  circle A678 centre (73.6938, -51.3062) radius 2.5
  circle A679 centre (80.5725, -45.1918) radius 2.5
  circle A680 centre (-66.3062, -45.3062) radius 2.5
  circle A681 centre (-59.4275, -39.1918) radius 2.5
  circle A682 centre (-59.3062, -45.3062) radius 2.5
  circle A683 centre (-52.4275, -39.1918) radius 2.5
  circle A684 centre (-52.3062, -45.3062) radius 2.5
  circle A685 centre (-45.4275, -39.1918) radius 2.5
  circle A686 centre (-45.3062, -45.3062) radius 2.5
  circle A687 centre (-38.4275, -39.1918) radius 2.5
  circle A688 centre (-38.3062, -45.3062) radius 2.5
  circle A689 centre (-31.4275, -39.1918) radius 2.5
  circle A690 centre (-31.3062, -45.3062) radius 2.5
  circle A691 centre (-24.4275, -39.1918) radius 2.5
  circle A692 centre (-24.3062, -45.3062) radius 2.5
  circle A693 centre (-17.4275, -39.1918) radius 2.5
  circle A694 centre (-17.3062, -45.3062) radius 2.5
  circle A695 centre (-10.4275, -39.1918) radius 2.5
  circle A696 centre (-10.3062, -45.3062) radius 2.5
  circle A697 centre (-3.4275, -39.1918) radius 2.5
  circle A698 centre (-3.3062, -45.3062) radius 2.5
  circle A699 centre (3.5725, -39.1918) radius 2.5
  circle A700 centre (3.6938, -45.3062) radius 2.5
  circle A701 centre (10.5725, -39.1918) radius 2.5
  circle A702 centre (10.6938, -45.3062) radius 2.5
  circle A703 centre (17.5725, -39.1918) radius 2.5
  circle A704 centre (17.6938, -45.3062) radius 2.5
  circle A705 centre (24.5725, -39.1918) radius 2.5
  circle A706 centre (24.6938, -45.3062) radius 2.5
  circle A707 centre (31.5725, -39.1918) radius 2.5
  circle A708 centre (31.6938, -45.3062) radius 2.5
  circle A709 centre (38.5725, -39.1918) radius 2.5
  circle A710 centre (38.6938, -45.3062) radius 2.5
  circle A711 centre (45.5725, -39.1918) radius 2.5
  circle A712 centre (45.6938, -45.3062) radius 2.5
  circle A713 centre (52.5725, -39.1918) radius 2.5
  circle A714 centre (52.6938, -45.3062) radius 2.5
  circle A715 centre (59.5725, -39.1918) radius 2.5
  circle A716 centre (59.6938, -45.3062) radius 2.5
  circle A717 centre (66.5725, -39.1918) radius 2.5
  circle A718 centre (66.6938, -45.3062) radius 2.5
  circle A719 centre (73.5725, -39.1918) radius 2.5
  circle A720 centre (73.6938, -45.3062) radius 2.5
  circle A721 centre (80.5725, -39.1918) radius 2.5
  circle A722 centre (-66.3062, -39.3062) radius 2.5
  circle A723 centre (-59.4275, -33.1918) radius 2.5
  circle A724 centre (-59.3062, -39.3062) radius 2.5
  circle A725 centre (-52.4275, -33.1918) radius 2.5
  circle A726 centre (-52.3062, -39.3062) radius 2.5
  circle A727 centre (-45.4275, -33.1918) radius 2.5
  circle A728 centre (-45.3062, -39.3062) radius 2.5
  circle A729 centre (-38.4275, -33.1918) radius 2.5
  circle A730 centre (-38.3062, -39.3062) radius 2.5
  circle A731 centre (-31.4275, -33.1918) radius 2.5
  circle A732 centre (-31.3062, -39.3062) radius 2.5
  circle A733 centre (-24.4275, -33.1918) radius 2.5
  circle A734 centre (-24.3062, -39.3062) radius 2.5
  circle A735 centre (-17.4275, -33.1918) radius 2.5
  circle A736 centre (-17.3062, -39.3062) radius 2.5
  circle A737 centre (-10.4275, -33.1918) radius 2.5
  circle A738 centre (-10.3062, -39.3062) radius 2.5
  circle A739 centre (-3.4275, -33.1918) radius 2.5
  circle A740 centre (-3.3062, -39.3062) radius 2.5
  circle A741 centre (3.5725, -33.1918) radius 2.5
  circle A742 centre (3.6938, -39.3062) radius 2.5
  circle A743 centre (10.5725, -33.1918) radius 2.5
  circle A744 centre (10.6938, -39.3062) radius 2.5
  circle A745 centre (17.5725, -33.1918) radius 2.5
  circle A746 centre (17.6938, -39.3062) radius 2.5
  circle A747 centre (24.5725, -33.1918) radius 2.5
  circle A748 centre (24.6938, -39.3062) radius 2.5
  circle A749 centre (31.5725, -33.1918) radius 2.5
  circle A750 centre (31.6938, -39.3062) radius 2.5
  circle A751 centre (38.5725, -33.1918) radius 2.5
  circle A752 centre (38.6938, -39.3062) radius 2.5
  circle A753 centre (45.5725, -33.1918) radius 2.5
  circle A754 centre (45.6938, -39.3062) radius 2.5
  circle A755 centre (52.5725, -33.1918) radius 2.5
  circle A756 centre (52.6938, -39.3062) radius 2.5
  circle A757 centre (59.5725, -33.1918) radius 2.5
  circle A758 centre (59.6938, -39.3062) radius 2.5
  circle A759 centre (66.5725, -33.1918) radius 2.5
  circle A760 centre (66.6938, -39.3062) radius 2.5
  circle A761 centre (73.5725, -33.1918) radius 2.5
  circle A762 centre (73.6938, -39.3062) radius 2.5
  circle A763 centre (80.5725, -33.1918) radius 2.5
  circle A764 centre (-66.3062, -33.3062) radius 2.5
  circle A765 centre (-59.4275, -27.1918) radius 2.5
  circle A766 centre (-59.3062, -33.3062) radius 2.5
  circle A767 centre (-52.4275, -27.1918) radius 2.5
  circle A768 centre (-52.3062, -33.3062) radius 2.5
  circle A769 centre (-45.4275, -27.1918) radius 2.5
  circle A770 centre (-45.3062, -33.3062) radius 2.5
  circle A771 centre (-38.4275, -27.1918) radius 2.5
  circle A772 centre (-38.3062, -33.3062) radius 2.5
  circle A773 centre (-31.4275, -27.1918) radius 2.5
  circle A774 centre (-31.3062, -33.3062) radius 2.5
  circle A775 centre (-24.4275, -27.1918) radius 2.5
  circle A776 centre (-24.3062, -33.3062) radius 2.5
  circle A777 centre (-17.4275, -27.1918) radius 2.5
  circle A778 centre (-17.3062, -33.3062) radius 2.5
  circle A779 centre (-10.4275, -27.1918) radius 2.5
  circle A780 centre (-10.3062, -33.3062) radius 2.5
  circle A781 centre (-3.4275, -27.1918) radius 2.5
  circle A782 centre (-3.3062, -33.3062) radius 2.5
  circle A783 centre (3.5725, -27.1918) radius 2.5
  circle A784 centre (3.6938, -33.3062) radius 2.5
  circle A785 centre (10.5725, -27.1918) radius 2.5
  circle A786 centre (10.6938, -33.3062) radius 2.5
  circle A787 centre (17.5725, -27.1918) radius 2.5
  circle A788 centre (17.6938, -33.3062) radius 2.5
  circle A789 centre (24.5725, -27.1918) radius 2.5
  circle A790 centre (24.6938, -33.3062) radius 2.5
  circle A791 centre (31.5725, -27.1918) radius 2.5
  circle A792 centre (31.6938, -33.3062) radius 2.5
  circle A793 centre (38.5725, -27.1918) radius 2.5
  circle A794 centre (38.6938, -33.3062) radius 2.5
  circle A795 centre (45.5725, -27.1918) radius 2.5
  circle A796 centre (45.6938, -33.3062) radius 2.5
  circle A797 centre (52.5725, -27.1918) radius 2.5
  circle A798 centre (52.6938, -33.3062) radius 2.5
  circle A799 centre (59.5725, -27.1918) radius 2.5
  circle A800 centre (59.6938, -33.3062) radius 2.5
  circle A801 centre (66.5725, -27.1918) radius 2.5
  circle A802 centre (66.6938, -33.3062) radius 2.5
  circle A803 centre (73.5725, -27.1918) radius 2.5
  circle A804 centre (73.6938, -33.3062) radius 2.5
  circle A805 centre (80.5725, -27.1918) radius 2.5
  circle A806 centre (-66.3062, -27.3062) radius 2.5
  circle A807 centre (-59.4275, -21.1918) radius 2.5
  circle A808 centre (-59.3062, -27.3062) radius 2.5
  circle A809 centre (-52.4275, -21.1918) radius 2.5
  circle A810 centre (-52.3062, -27.3062) radius 2.5
  circle A811 centre (-45.4275, -21.1918) radius 2.5
  circle A812 centre (-45.3062, -27.3062) radius 2.5
  circle A813 centre (-38.4275, -21.1918) radius 2.5
  circle A814 centre (-38.3062, -27.3062) radius 2.5
  circle A815 centre (-31.4275, -21.1918) radius 2.5
  circle A816 centre (-31.3062, -27.3062) radius 2.5
  circle A817 centre (-24.4275, -21.1918) radius 2.5
  circle A818 centre (-24.3062, -27.3062) radius 2.5
  circle A819 centre (-17.4275, -21.1918) radius 2.5
  circle A820 centre (-17.3062, -27.3062) radius 2.5
  circle A821 centre (-10.4275, -21.1918) radius 2.5
  circle A822 centre (-10.3062, -27.3062) radius 2.5
  circle A823 centre (-3.4275, -21.1918) radius 2.5
  circle A824 centre (-3.3062, -27.3062) radius 2.5
  circle A825 centre (3.5725, -21.1918) radius 2.5
  circle A826 centre (3.6938, -27.3062) radius 2.5
  circle A827 centre (10.5725, -21.1918) radius 2.5
  circle A828 centre (10.6938, -27.3062) radius 2.5
  circle A829 centre (17.5725, -21.1918) radius 2.5
  circle A830 centre (17.6938, -27.3062) radius 2.5
  circle A831 centre (24.5725, -21.1918) radius 2.5
  circle A832 centre (24.6938, -27.3062) radius 2.5
  circle A833 centre (31.5725, -21.1918) radius 2.5
  circle A834 centre (31.6938, -27.3062) radius 2.5
  circle A835 centre (38.5725, -21.1918) radius 2.5
  circle A836 centre (38.6938, -27.3062) radius 2.5
  circle A837 centre (45.5725, -21.1918) radius 2.5
  circle A838 centre (45.6938, -27.3062) radius 2.5
  circle A839 centre (52.5725, -21.1918) radius 2.5
  circle A840 centre (52.6938, -27.3062) radius 2.5
  circle A841 centre (59.5725, -21.1918) radius 2.5
  circle A842 centre (59.6938, -27.3062) radius 2.5
  circle A843 centre (66.5725, -21.1918) radius 2.5
  circle A844 centre (66.6938, -27.3062) radius 2.5
  circle A845 centre (73.5725, -21.1918) radius 2.5
  circle A846 centre (73.6938, -27.3062) radius 2.5
  circle A847 centre (80.5725, -21.1918) radius 2.5
  circle A848 centre (-66.3062, -21.3062) radius 2.5
  circle A849 centre (-59.4275, -15.1918) radius 2.5
  circle A850 centre (-59.3062, -21.3062) radius 2.5
  circle A851 centre (-52.4275, -15.1918) radius 2.5
  circle A852 centre (-52.3062, -21.3062) radius 2.5
  circle A853 centre (-45.4275, -15.1918) radius 2.5
  circle A854 centre (-45.3062, -21.3062) radius 2.5
  circle A855 centre (-38.4275, -15.1918) radius 2.5
  circle A856 centre (-38.3062, -21.3062) radius 2.5
  circle A857 centre (-31.4275, -15.1918) radius 2.5
  circle A858 centre (-31.3062, -21.3062) radius 2.5
  circle A859 centre (-24.4275, -15.1918) radius 2.5
  circle A860 centre (-24.3062, -21.3062) radius 2.5
  circle A861 centre (-17.4275, -15.1918) radius 2.5
  circle A862 centre (-17.3062, -21.3062) radius 2.5
  circle A863 centre (-10.4275, -15.1918) radius 2.5
  circle A864 centre (-10.3062, -21.3062) radius 2.5
  circle A865 centre (-3.4275, -15.1918) radius 2.5
  circle A866 centre (-3.3062, -21.3062) radius 2.5
  circle A867 centre (3.5725, -15.1918) radius 2.5
  circle A868 centre (3.6938, -21.3062) radius 2.5
  circle A869 centre (10.5725, -15.1918) radius 2.5
  circle A870 centre (10.6938, -21.3062) radius 2.5
  circle A871 centre (17.5725, -15.1918) radius 2.5
  circle A872 centre (17.6938, -21.3062) radius 2.5
  circle A873 centre (24.5725, -15.1918) radius 2.5
  circle A874 centre (24.6938, -21.3062) radius 2.5
  circle A875 centre (31.5725, -15.1918) radius 2.5
  circle A876 centre (31.6938, -21.3062) radius 2.5
  circle A877 centre (38.5725, -15.1918) radius 2.5
  circle A878 centre (38.6938, -21.3062) radius 2.5
  circle A879 centre (45.5725, -15.1918) radius 2.5
  circle A880 centre (45.6938, -21.3062) radius 2.5
  circle A881 centre (52.5725, -15.1918) radius 2.5
  circle A882 centre (52.6938, -21.3062) radius 2.5
  circle A883 centre (59.5725, -15.1918) radius 2.5
  circle A884 centre (59.6938, -21.3062) radius 2.5
  circle A885 centre (66.5725, -15.1918) radius 2.5
  circle A886 centre (66.6938, -21.3062) radius 2.5
  circle A887 centre (73.5725, -15.1918) radius 2.5
  circle A888 centre (73.6938, -21.3062) radius 2.5
  circle A889 centre (80.5725, -15.1918) radius 2.5
  circle A890 centre (-66.3062, -15.3062) radius 2.5
  circle A891 centre (-59.4275, -9.1918) radius 2.5
  circle A892 centre (-59.3062, -15.3062) radius 2.5
  circle A893 centre (-52.4275, -9.1918) radius 2.5
  circle A894 centre (-52.3062, -15.3062) radius 2.5
  circle A895 centre (-45.4275, -9.1918) radius 2.5
  circle A896 centre (-45.3062, -15.3062) radius 2.5
  circle A897 centre (-38.4275, -9.1918) radius 2.5
  circle A898 centre (-38.3062, -15.3062) radius 2.5
  circle A899 centre (-31.4275, -9.1918) radius 2.5
  circle A900 centre (-31.3062, -15.3062) radius 2.5
  circle A901 centre (-24.4275, -9.1918) radius 2.5
  circle A902 centre (-24.3062, -15.3062) radius 2.5
  circle A903 centre (-17.4275, -9.1918) radius 2.5
  circle A904 centre (-17.3062, -15.3062) radius 2.5
  circle A905 centre (-10.4275, -9.1918) radius 2.5
  circle A906 centre (-10.3062, -15.3062) radius 2.5
  circle A907 centre (-3.4275, -9.1918) radius 2.5
  circle A908 centre (-3.3062, -15.3062) radius 2.5
  circle A909 centre (3.5725, -9.1918) radius 2.5
  circle A910 centre (3.6938, -15.3062) radius 2.5
  circle A911 centre (10.5725, -9.1918) radius 2.5
  circle A912 centre (10.6938, -15.3062) radius 2.5
  circle A913 centre (17.5725, -9.1918) radius 2.5
  circle A914 centre (17.6938, -15.3062) radius 2.5
  circle A915 centre (24.5725, -9.1918) radius 2.5
  circle A916 centre (24.6938, -15.3062) radius 2.5
  circle A917 centre (31.5725, -9.1918) radius 2.5
  circle A918 centre (31.6938, -15.3062) radius 2.5
  circle A919 centre (38.5725, -9.1918) radius 2.5
  circle A920 centre (38.6938, -15.3062) radius 2.5
  circle A921 centre (45.5725, -9.1918) radius 2.5
  circle A922 centre (45.6938, -15.3062) radius 2.5
  circle A923 centre (52.5725, -9.1918) radius 2.5
  circle A924 centre (52.6938, -15.3062) radius 2.5
  circle A925 centre (59.5725, -9.1918) radius 2.5
  circle A926 centre (59.6938, -15.3062) radius 2.5
  circle A927 centre (66.5725, -9.1918) radius 2.5
  circle A928 centre (66.6938, -15.3062) radius 2.5